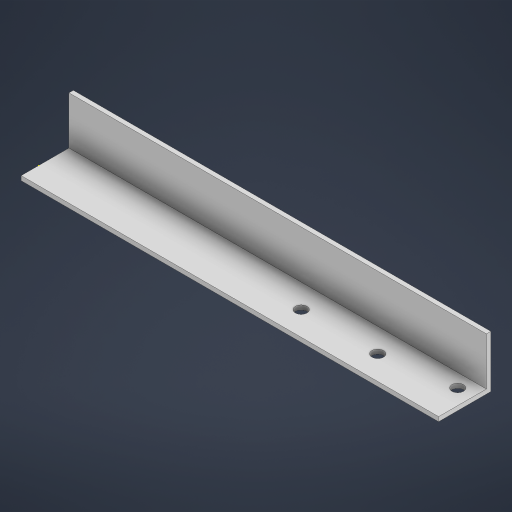
# Autodesk Inventor part: wing
Saved by Autodesk Inventor 2024 (Build 280153000, 153)
## iProperties
Created: 2023-12-24
Part Number: wing
Material: Generic
Document SubType Name: Modeling
Designer: elite
Density: 1 g/cm^3
Appearance: Default
Author: elite
Autodesk Inventor part; units mm, degrees
ref_plane "YZ Plane" through (0, 0, 0) normal (1, 0, 0) x (0, 1, 0)
ref_plane "XZ Plane" through (0, 0, 0) normal (0, 1, 0) x (-1, 0, 0)
ref_plane "XY Plane" through (0, 0, 0) normal (0, 0, 1) x (1, 0, 0)
sketch "Sketch1" plane through (0, 0, 0) normal (1, 0, 0) x (0, 1, 0)
  line L0 (0, 0) -> (1.6002, 0)
  line L1 (1.6002, 0) -> (1.6002, -12.7)
  line L2 (1.6002, -12.7) -> (0, -12.7)
  line L3 (0, -12.7) -> (0, 0)
  line L4 (0, -12.7) -> (0, -11.0998)
  line L5 (0, -11.0998) -> (12.7, -11.0998)
  line L6 (12.7, -11.0998) -> (12.7, -12.7)
  line L7 (12.7, -12.7) -> (0, -12.7)
  line L8 (0, -12.7) -> (0, -11.0998)
  point P0 (1.6002, -11.0998)
  dimension "d0" = 1.6002
  dimension "d1" = 12.7
  dimension "d2" = 1.6002
  dimension "d3" = 12.7
  constraints: 18 end point, 4 parallel, 2 horizontal, 2 perpendicular, 2 point on line
  measures "d0" distance of L1.end L2.end
  measures "d1" distance of L2.end L0.start
  measures "d2" distance of L2.end L4.end
  measures "d3" distance of L6.end L7.end
extrude "Extrusion1" add sketch "Sketch1" along normal blind 152.4
sketch "Sketch4" plane through (0, 0, 0) normal (0, 0, 1) x (1, 0, 0)
  line L0 (0, 1.6002) -> (152.4, 1.6002) projected
  line L1 (0, 0) -> (152.4, 0)
  line L2 (152.4, 0) -> (152.4, 1.6002)
  line L3 (152.4, 1.6002) -> (0, 1.6002)
  line L4 (0, 1.6002) -> (0, 0)
  constraints: 8 end point, 2 parallel, 1 horizontal, 1 perpendicular
extrude "Extrusion4" add sketch "Sketch4" along normal blind 6.35
sketch "Sketch5" plane through (0, 12.7, -11.0998) normal (0, 1, 0) x (1, 0, 0)
  line L0 (0, 0) -> (152.4, 0) projected
  line L1 (152.4, 1.6002) -> (152.4, -17.4498) projected
  line L2 (0, 0) -> (152.4, 0)
  line L3 (152.4, 0) -> (152.4, 1.6002)
  line L4 (152.4, 1.6002) -> (0, 1.6002)
  line L5 (0, 1.6002) -> (0, 0)
  point P0 (0, -11.0998)
  constraints: 8 end point, 2 parallel, 1 horizontal, 1 perpendicular
extrude "Extrusion5" add sketch "Sketch5" along normal blind 6.35
sketch "Sketch6" plane through (0, 1.6002, -11.0998) normal (0, 1, 0) x (1, 0, 0)
  point P0 (0, -11.0998)
sketch "Sketch7" plane through (0, 1.6002, -11.0998) normal (0, 1, 0) x (1, 0, 0)
  line L0 (152.4, 1.6002) -> (152.4, -17.4498) projected
  line L1 (152.4, -17.4498) -> (152.4, 0.0127)
  line L2 (152.4, -8.7185) -> (146.8374, -8.7185)
  line L3 (146.8374, -8.7185) -> (121.4374, -8.7185)
  circle A0 centre (121.4374, -8.7185) radius 2.1082
  line L4 (121.4374, -8.7185) -> (93.4974, -8.7186)
  circle A1 centre (93.4974, -8.7186) radius 2.1082
  line L5 (146.8374, -8.7185) -> (146.8374, -4.9085)
  circle A2 centre (146.8374, -4.9085) radius 2.1082
  point P0 (0, -11.0998)
  dimension "d19" = 17.4625
  dimension "d20" = 5.5626
  dimension "d22" = 25.4
  dimension "d23" = 27.94
  dimension "d24" = 4.2164
  dimension "d27" = 3.81
  dimension "d28" = 4.2164
  constraints: 10 end point, 4 coincident, 3 centre point, 3 horizontal, 1 midpoint, 1 point on line, 1 vertical
  measures "d19" distance of L0.end L1.end
  measures "d20" distance of L2.start L2.end
  measures "d22" distance of L3.start L3.end
  measures "d23" distance of L4.start L4.end
  measures "d24" diameter of A1
  measures "d27" distance of L3.start L5.end
  measures "d28" diameter of A2
extrude "Extrusion6" cut sketch "Sketch7" against normal blind 25.4
body "Solid1"
